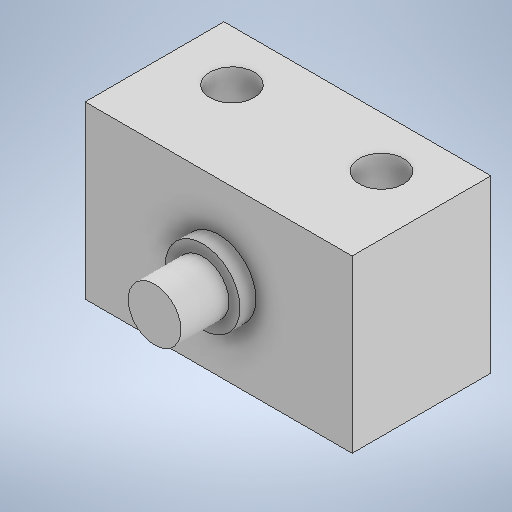
# Autodesk Inventor part: 13042026-03
Saved by Autodesk Inventor 2025.2 (Build 292293000, 293)
## iProperties
Created: 2026-05-05
Part Number: 13042026-03
Material: Generic
Document SubType Name: Modeling
Designer: Oski
Density: 1 g/cm^3
Appearance: Default
Author: Oski
Autodesk Inventor part; units mm, degrees
ref_plane "YZ Plane" through (0, 0, 0) normal (1, 0, 0) x (0, 1, 0)
ref_plane "XZ Plane" through (0, 0, 0) normal (0, 1, 0) x (-1, 0, 0)
ref_plane "XY Plane" through (0, 0, 0) normal (0, 0, 1) x (1, 0, 0)
sketch "Sketch2" plane through (0, 0, 0) normal (0, 0, 1) x (1, 0, 0)
  line L0 (-25, 16) -> (25, 16)
  line L1 (25, 16) -> (25, -16)
  line L2 (25, -16) -> (-25, -16)
  line L3 (-25, -16) -> (-25, 16)
  line L4 (-25, 16) -> (25, -16) construction
  line L5 (25, 16) -> (-25, -16) construction
  point P0 (0, 0)
  dimension "d4" = 32
  dimension "d5" = 50
  constraints: 12 end point, 2 midpoint, 2 parallel, 1 horizontal, 1 perpendicular
  measures "d4" distance of L0.end L1.end
  measures "d5" distance of L1.end L2.end
extrude "Extrusion1" add sketch "Sketch2" along normal blind 26
sketch "Sketch3" plane through (0, 0, 26) normal (0, 0, 1) x (1, 0, 0)
  circle A0 centre (0, 0) radius 7
  dimension "d8" = 14
  constraints: 1 centre point, 1 coincident
  measures "d8" diameter of A0
extrude "Extrusion2" add sketch "Sketch3" along normal blind 3
sketch "Sketch4" plane through (0, 0, 29) normal (0, 0, 1) x (1, 0, 0)
  circle A0 centre (0, 0) radius 4.95
  dimension "d11" = 9.9
  constraints: 1 centre point, 1 coincident
  measures "d11" diameter of A0
extrude "Extrusion3" add sketch "Sketch4" along normal blind 9
sketch "Sketch6" plane through (-25, 16, 0) normal (0, 1, 0) x (1, 0, 0)
  line L0 (11, -9.5) -> (0, -9.5) construction
  line L1 (0, 0) -> (0, -26) projected
  line L2 (39, -9.5) -> (50, -9.5) construction
  line L3 (50, 0) -> (50, -26) projected
  line L4 (50, 0) -> (0, 0) projected
  point P0 (25, 0)
  point P1 (44.5, -9.5)
  dimension "d29" = 28
  dimension "d30" = 9.5
  constraints: 4 end point, 3 point on line, 2 horizontal, 1 collinear, 1 midpoint
  measures "d29" distance of L2.start L0.start
  measures "d30" distance from line of L4 point (44.5, -9.5)
hole "Hole3" at (-14, 16, 9.5) at (14, 16, 9.5) direction (0, -1, 0) diameter 8.3 end through all
body "Solid1"
